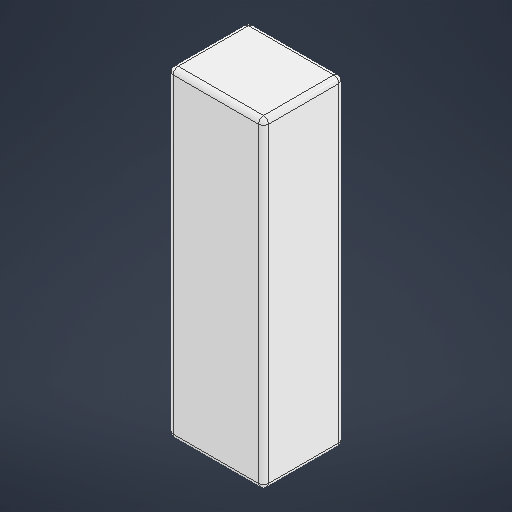
# Autodesk Inventor part: Schussakku
Saved by Autodesk Inventor 2025.2 (Build 292293000, 293)
## iProperties
Created: 2024-05-04
Part Number: Schussakku
Material: Generisch
Document SubType Name: Modeling
Designer: Fabian
Density: 1 g/cm^3
Appearance: Weiß
Author: Fabian
Autodesk Inventor part; units mm, degrees
ref_plane "YZ Plane" through (0, 0, 0) normal (1, 0, 0) x (0, 1, 0)
ref_plane "XZ Plane" through (0, 0, 0) normal (0, 1, 0) x (-1, 0, 0)
ref_plane "XY Plane" through (0, 0, 0) normal (0, 0, 1) x (1, 0, 0)
sketch "Skizze1" plane through (0, 0, 0) normal (0, 1, 0) x (-1, 0, 0)
  line L0 (-9.5, 8) -> (9.5, 8)
  line L1 (9.5, 8) -> (9.5, -8)
  line L2 (9.5, -8) -> (-9.5, -8)
  line L3 (-9.5, -8) -> (-9.5, 8)
  line L4 (-9.5, 8) -> (9.5, -8) construction
  line L5 (9.5, 8) -> (-9.5, -8) construction
  point P0 (0, 0)
  dimension "d0" = 19
  dimension "d1" = 16
  constraints: 12 end point, 2 midpoint, 2 parallel, 1 horizontal, 1 perpendicular
  measures "d0" distance of L1.end L2.end
  measures "d1" distance of L0.end L1.end
extrude "Extrusion1" add sketch "Skizze1" along normal blind 64
fillet "Rundung1" radius 1 12 edges at (9.5, 32, 8) (-9.5, 32, 8) (-9.5, 32, -8) (9.5, 32, -8) (9.5, 64, 0) (0, 64, 8) (-9.5, 64, 0) (0, 64, -8) (9.5, 0, 0) (0, 0, 8) (0, 0, -8) (-9.5, 0, 0)
